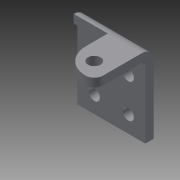
# Autodesk Inventor part: Clamp Piston Left Mount
Saved by Autodesk Inventor 2014 (Build 180170000, 170)
## iProperties
Created: 2014-02-22
Part Number: Clamp Piston Left Mount
Material: Generic
Document SubType Name: Sheet Metal
Designer: Michael
Density: 1 g/cm^3
Flat Pattern Width: 4.73693 cm
Flat Pattern Length: 2.54 cm
Flat Pattern Area: 12.0318 cm^2
Sheet Metal Rule: Default
Sheet Metal Width: 1.865 in
Sheet Metal Length: 1.000 in
Sheet Metal Area: 1.865 in^2
Appearance: Default
Author: Michael
Autodesk Inventor part; units mm, degrees
ref_plane "YZ Plane" through (0, 0, 0) normal (1, 0, 0) x (0, 1, 0)
ref_plane "XZ Plane" through (0, 0, 0) normal (0, 1, 0) x (-1, 0, 0)
ref_plane "XY Plane" through (0, 0, 0) normal (0, 0, 1) x (1, 0, 0)
sketch "Sketch1" plane through (0, 0, 0) normal (0, 0, 1) x (1, 0, 0)
  line L0 (0, 0) -> (25.4, 0)
  line L1 (25.4, 0) -> (25.4, 25.4)
  line L2 (25.4, 25.4) -> (0, 25.4)
  line L3 (0, 25.4) -> (0, 0)
  circle A0 centre (6.35, 19.05) radius 2.0828
  circle A1 centre (19.05, 19.05) radius 2.0828
  circle A2 centre (6.35, 6.35) radius 2.0828
  circle A3 centre (19.05, 6.35) radius 2.0828
  dimension "d0" = 25.4
  dimension "d1" = 25.4
  dimension "d2" = 4.1656
  dimension "d3" = 6.35
  dimension "d4" = 6.35
  dimension "d7" = 12.7
  dimension "d10" = 12.7
  measures "d0" distance of L2.end L1.end
  measures "d1" distance of L1.end L0.end
  measures "d2" diameter of A0
  measures "d3" distance from line of L2 A0.centre
  measures "d4" distance from line of L3 A0.centre
  measures "d7" distance of A0.centre A1.centre
  measures "d10" distance of A0.centre A2.centre
extrude "Plate1" add sketch "Sketch1" along normal blind 3.175
sketch "Sketch2" plane through (0, 26.67, 4.445) normal (0, 1, 0) x (-1, 0, 0)
  line L0 (-25.4, 0) -> (0, 0)
  line L1 (0, 0) -> (0, 17.78)
  line L2 (0, 17.78) -> (-25.4, 17.78)
  line L3 (-25.4, 17.78) -> (-25.4, 0)
  constraints: 6 end point, 1 horizontal, 1 perpendicular, 1 vertical
edge flange "Flange1" height 22.225 angle 90 thickness 3.175 bend radius 1.27 thickness toward (0, 1, 0) relief straight relief width 3.175 relief depth 1.5875 edges at (12.7, 25.4, 3.175) wall of the first edge with corners at (25.4, 26.67, 4.445) (0, 26.67, 4.445) (0, 26.67, 22.225) (25.4, 26.67, 22.225)
bend "Bend1"
corner "Corner1"
sketch "Sketch3" plane through (0, 29.845, 22.225) normal (0, 1, 0) x (1, 0, 0)
  line L0 (25.4, 17.78) -> (0, 17.78) projected
  line L1 (0, 0) -> (0, 17.78) projected
  line L2 (25.4, 0) -> (0, 0) projected
  line L3 (25.4, 17.78) -> (25.4, 0) projected
  line L4 (25.4, 0) -> (0, 0)
  line L5 (25.4, 17.78) -> (25.4, 0)
  circle A0 centre (19.05, 6.35) radius 2.3749
  line L6 (0, 0) -> (0, 20.955)
  line L7 (25.4, 17.78) -> (0, 17.78)
  line L8 (12.7, 17.78) -> (12.7, 9.525)
  arc A1 (12.7, 9.525) -> (22.225, 0) centre (22.225, 9.525) ccw
  arc A2 (12.7, 9.525) -> (22.225, 0) centre (22.225, 9.525) ccw
  line L9 (12.7, 9.525) -> (12.7, 17.78)
  line L10 (12.7, 17.78) -> (25.4, 17.78)
  line L11 (25.4, 17.78) -> (25.4, 0)
  line L12 (25.4, 0) -> (22.225, 0)
  point P0 (0, 22.225)
  dimension "d24" = 4.7498
  dimension "d25" = 6.35
  dimension "d26" = 6.35
  dimension "d27" = 9.525
  dimension "d28" = 3.175
  dimension "d29" = 12.7
  constraints: 18 end point, 6 collinear, 5 tangent, 4 point on circle, 3 centre point, 1 concentric, 1 midpoint, 1 perpendicular, 1 point on line, 1 vertical
  measures "d24" diameter of A0
  measures "d25" horizontal distance of L11.end A0.centre
  measures "d26" distance from line of L2 A0.centre
  measures "d27" radius of A1
  measures "d28" distance from line of L3 L12.end
  measures "d29" distance from line of L3 L8.start
extrude "Extrusion1" cut sketch "Sketch3" against normal blind 25.4 contours L8 A1 L2 L1 L0 | A0
fillet "Fillet1" radius 3.175 1 edges at (25.4, 28.2575, 22.225)
equation "\"d14\" = BendReliefWidth"
equation "\"d15\" = BendReliefDepth"
equation "\"d16\" = MinimumRemnant"
equation "\"d17\" = BendRadius"
equation "\"d21\" = CornerReliefSize"
equation "\"d22\" = GapSize"
equation "\"d23\" = JacobiRadiusSize"
equation "\"BendRadius\" = Thickness"
equation "\"BendReliefWidth\" = Thickness"
equation "\"BendReliefDepth\" = 0.5 * Thickness"
equation "\"CornerReliefSize\" = 4 * Thickness"
equation "\"MinimumRemnant\" = 2 * Thickness"
equation "\"TransitionRadius\" = BendRadius"
equation "\"JacobiRadiusSize\" = BendRadius"
equation "\"GapSize\" = Thickness"
equation "\"d13\" = BendRadius"
equation "\"Thickness\" = 3.175"
body "Solid1"
